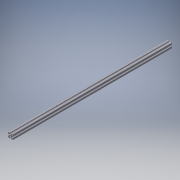
# Autodesk Inventor part: 30x30-01
Saved by Autodesk Inventor 2016 SP1 (Build 200210100, 210)
## iProperties
Created: 2005-12-12
Part Number: 30x30-01
Document SubType Name: Modeling
Designer: Administrator
Material: Aluminum-6061
Description: PROFILE 30X30
Stock Number: 20.1068 PROFILE 30X30
Density: 2.71 g/cm^3
Appearance: Aluminum - Flat
FINISH: CLEAR ANODIZED
Author: Administrator
Autodesk Inventor part; units mm, degrees
ref_plane "YZ Plane" through (0, 0, 0) normal (1, 0, 0) x (0, 1, 0)
ref_plane "XZ Plane" through (0, 0, 0) normal (0, 1, 0) x (-1, 0, 0)
ref_plane "XY Plane" through (0, 0, 0) normal (0, 0, 1) x (1, 0, 0)
sketch "Sketch1" plane through (0, 0, 0) normal (0, 0, 1) x (1, 0, 0)
  arc A0 (9.3, -7.8) -> (7.8, -9.3) centre (9.3, -9.3) ccw
  line L0 (13.5, -7.8) -> (9.3, -7.8)
  arc A1 (14, -8.3) -> (13.5, -7.8) centre (13.5, -8.3) ccw
  line L1 (14, -12.5) -> (14, -8.3)
  arc A2 (12.5, -14) -> (14, -12.5) centre (12.5, -12.5) ccw
  line L2 (8.3, -14) -> (12.5, -14)
  arc A3 (7.8, -13.5) -> (8.3, -14) centre (8.3, -13.5) ccw
  line L3 (7.8, -9.3) -> (7.8, -13.5)
  arc A4 (-13.5, -7.8) -> (-14, -8.3) centre (-13.5, -8.3) ccw
  line L4 (-9.3, -7.8) -> (-13.5, -7.8)
  arc A5 (-7.8, -9.3) -> (-9.3, -7.8) centre (-9.3, -9.3) ccw
  line L5 (-7.8, -13.5) -> (-7.8, -9.3)
  arc A6 (-8.3, -14) -> (-7.8, -13.5) centre (-8.3, -13.5) ccw
  line L6 (-12.5, -14) -> (-8.3, -14)
  arc A7 (-14, -12.5) -> (-12.5, -14) centre (-12.5, -12.5) ccw
  line L7 (-14, -8.3) -> (-14, -12.5)
  line L8 (3.2859, 3.8789) -> (2.2431, 3.6573)
  arc A8 (3.8789, 3.2859) -> (3.2859, 3.8789) centre (3.3898, 3.3898) ccw
  line L9 (3.6573, 2.2431) -> (3.8789, 3.2859)
  line L10 (3.2627, 1.8485) -> (3.6573, 2.2431)
  line L11 (3.6573, -2.2431) -> (3.2627, -1.8485)
  line L12 (3.8789, -3.2859) -> (3.6573, -2.2431)
  arc A9 (3.2859, -3.8789) -> (3.8789, -3.2859) centre (3.3898, -3.3898) ccw
  line L13 (2.2431, -3.6573) -> (3.2859, -3.8789)
  line L14 (1.8485, -3.2627) -> (2.2431, -3.6573)
  arc A10 (-1.8485, -3.2627) -> (1.6602, -3.3625) centre (0, 0) ccw
  line L15 (-2.2431, -3.6573) -> (-1.8485, -3.2627)
  line L16 (-3.2859, -3.8789) -> (-2.2431, -3.6573)
  arc A11 (-3.8789, -3.2859) -> (-3.2859, -3.8789) centre (-3.3898, -3.3898) ccw
  line L17 (-3.6573, -2.2431) -> (-3.8789, -3.2859)
  line L18 (-3.2627, -1.8485) -> (-3.6573, -2.2431)
  arc A12 (-3.3625, 1.6602) -> (-3.2627, -1.8485) centre (0, 0) ccw
  line L19 (-3.6573, 2.2431) -> (-3.2627, 1.8485)
  line L20 (-3.8789, 3.2859) -> (-3.6573, 2.2431)
  arc A13 (-3.2859, 3.8789) -> (-3.8789, 3.2859) centre (-3.3898, 3.3898) ccw
  line L21 (-2.2431, 3.6573) -> (-3.2859, 3.8789)
  line L22 (-1.8485, 3.2627) -> (-2.2431, 3.6573)
  line L23 (2.2431, 3.6573) -> (1.8485, 3.2627)
  arc A14 (13.5, 7.8) -> (14, 8.3) centre (13.5, 8.3) ccw
  line L24 (9.3, 7.8) -> (13.5, 7.8)
  arc A15 (7.8, 9.3) -> (9.3, 7.8) centre (9.3, 9.3) ccw
  line L25 (7.8, 13.5) -> (7.8, 9.3)
  arc A16 (8.3, 14) -> (7.8, 13.5) centre (8.3, 13.5) ccw
  line L26 (12.5, 14) -> (8.3, 14)
  arc A17 (14, 12.5) -> (12.5, 14) centre (12.5, 12.5) ccw
  line L27 (14, 8.3) -> (14, 12.5)
  arc A18 (-12.5, 14) -> (-14, 12.5) centre (-12.5, 12.5) ccw
  line L28 (-8.3, 14) -> (-12.5, 14)
  arc A19 (-7.8, 13.5) -> (-8.3, 14) centre (-8.3, 13.5) ccw
  line L29 (-7.8, 9.3) -> (-7.8, 13.5)
  arc A20 (-9.3, 7.8) -> (-7.8, 9.3) centre (-9.3, 9.3) ccw
  line L30 (-13.5, 7.8) -> (-9.3, 7.8)
  arc A21 (-14, 8.3) -> (-13.5, 7.8) centre (-13.5, 8.3) ccw
  line L31 (-14, 12.5) -> (-14, 8.3)
  line L32 (12.5, 4.1) -> (12.5, 6.8)
  line L33 (15, 4.1) -> (12.5, 4.1)
  line L34 (15, 15) -> (15, 4.1)
  line L35 (4.1, 15) -> (15, 15)
  line L36 (4.1, 12.5) -> (4.1, 15)
  line L37 (6.8, 12.5) -> (4.1, 12.5)
  line L38 (6.8, 7.8606) -> (6.8, 12.5)
  line L39 (3.9715, 5.0321) -> (6.8, 7.8606)
  line L40 (-3.9715, 5.0321) -> (3.9715, 5.0321)
  line L41 (-6.8, 7.8606) -> (-3.9715, 5.0321)
  line L42 (-6.8, 12.5) -> (-6.8, 7.8606)
  line L43 (-4.1, 12.5) -> (-6.8, 12.5)
  line L44 (-4.1, 15) -> (-4.1, 12.5)
  line L45 (-15, 15) -> (-4.1, 15)
  line L46 (-15, 4.1) -> (-15, 15)
  line L47 (-12.5, 4.1) -> (-15, 4.1)
  line L48 (-12.5, 6.8) -> (-12.5, 4.1)
  line L49 (-7.8606, 6.8) -> (-12.5, 6.8)
  line L50 (-5.0321, 3.9715) -> (-7.8606, 6.8)
  line L51 (-5.0321, -3.9715) -> (-5.0321, 3.9715)
  line L52 (-7.8606, -6.8) -> (-5.0321, -3.9715)
  line L53 (-12.5, -6.8) -> (-7.8606, -6.8)
  line L54 (-12.5, -4.1) -> (-12.5, -6.8)
  line L55 (-15, -4.1) -> (-12.5, -4.1)
  line L56 (-15, -15) -> (-15, -4.1)
  line L57 (-4.1, -15) -> (-15, -15)
  line L58 (-4.1, -12.5) -> (-4.1, -15)
  line L59 (-6.8, -12.5) -> (-4.1, -12.5)
  line L60 (-6.8, -7.8606) -> (-6.8, -12.5)
  line L61 (-3.9715, -5.0321) -> (-6.8, -7.8606)
  line L62 (3.9715, -5.0321) -> (-3.9715, -5.0321)
  line L63 (6.8, -7.8606) -> (3.9715, -5.0321)
  line L64 (6.8, -12.5) -> (6.8, -7.8606)
  line L65 (4.1, -12.5) -> (6.8, -12.5)
  line L66 (4.1, -15) -> (4.1, -12.5)
  line L67 (15, -15) -> (4.1, -15)
  line L68 (15, -4.1) -> (15, -15)
  line L69 (12.5, -4.1) -> (15, -4.1)
  line L70 (12.5, -6.8) -> (12.5, -4.1)
  line L71 (7.8606, -6.8) -> (12.5, -6.8)
  line L72 (5.0321, -3.9715) -> (7.8606, -6.8)
  line L73 (5.0321, 3.9715) -> (5.0321, -3.9715)
  line L74 (7.8606, 6.8) -> (5.0321, 3.9715)
  line L75 (12.5, 6.8) -> (7.8606, 6.8)
  arc A22 (-3.2627, 1.8485) -> (-3.3625, 1.6602) centre (0, 0) ccw
  arc A23 (3.3625, 1.6602) -> (3.2627, 1.8485) centre (0, 0) ccw
  arc A24 (1.8485, 3.2627) -> (-1.8485, 3.2627) centre (0, 0) ccw
  arc A25 (1.6602, -3.3625) -> (1.8485, -3.2627) centre (0, 0) ccw
  arc A26 (3.2627, -1.8485) -> (3.3625, 1.6602) centre (0, 0) ccw
  constraints: 152 end point, 54 point on circle, 27 centre point, 26 horizontal, 26 vertical, 179 other
extrude "Extrusion1" add sketch "Sketch1" along normal blind 1000
body "Solid1"
